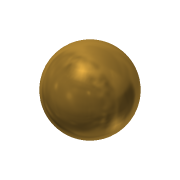
# Autodesk Inventor part: Brassweight
Saved by Autodesk Inventor 2016 (Build 200138000, 138)
## iProperties
Created: 2015-05-20
Part Number: Brassweight
Material: Brass, Soft Yellow
Document SubType Name: Modeling
Designer: Andy
Mass: 136.8 g
Surface Area: 26.4208 cm^2
Volume: 12.7701 cm^3
Density: 10.7126 g/cm^3
Appearance: Brass - Satin
Author: Andy
Autodesk Inventor part; units mm, degrees
ref_plane "YZ Plane" through (0, 0, 0) normal (1, 0, 0) x (0, 1, 0)
ref_plane "XZ Plane" through (0, 0, 0) normal (0, 1, 0) x (-1, 0, 0)
ref_plane "XY Plane" through (0, 0, 0) normal (0, 0, 1) x (1, 0, 0)
sketch "Sketch1" plane through (0, 0, 0) normal (1, 0, 0) x (0, 1, 0)
  arc A0 (-1.8, 14.5) -> (-1.8, -14.5) centre (-1.8, 0) ccw
  line L0 (-1.8, 14.5) -> (-1.8, -14.5)
  point P0 (0, 0)
  point P1 (-16.3, 0)
  dimension "d0" = 90
  constraints: 2 end point, 2 point on circle, 1 centre point, 1 coincident, 1 midpoint, 1 vertical
revolve "Revolution1" add sketch "Sketch1" angle 360 about axis through (0, -1.8, 14.5) along (0, 0, -1)
body "Solid1"
